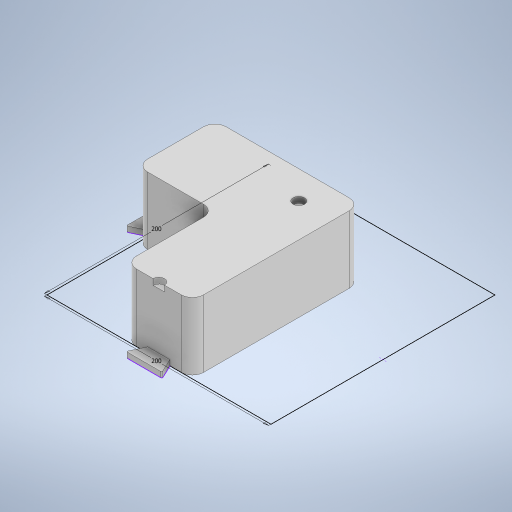
# Autodesk Inventor part: Area øv1
Saved by Autodesk Inventor 2024 (Build 280153000, 153)
## iProperties
Created: 2024-03-01
Part Number: Area øv1
Material: Generic
Document SubType Name: Modeling
Designer: laura
Density: 1 g/cm^3
Appearance: Default
Author: laura
Autodesk Inventor part; units mm, degrees
ref_plane "YZ Plane" through (0, 0, 0) normal (1, 0, 0) x (0, 1, 0)
ref_plane "XZ Plane" through (0, 0, 0) normal (0, 1, 0) x (-1, 0, 0)
ref_plane "XY Plane" through (0, 0, 0) normal (0, 0, 1) x (1, 0, 0)
sketch "Sketch1" plane through (0, 0, 0) normal (0, 1, 0) x (-1, 0, 0)
  line L0 (0, 0) -> (200, 0)
  line L1 (200, 0) -> (200, 200)
  line L2 (200, 200) -> (0, 200)
  line L3 (0, 200) -> (0, 0)
  line L4 (110, 199.8) -> (110, 213.2303) construction
  line L5 (100, 213.1946) -> (114.7696, 213.1946)
  arc A0 (115.4946, 212.0565) -> (114.7696, 213.1946) centre (114.7696, 212.3946) ccw
  line L6 (115.4946, 212.0565) -> (109.8726, 200)
  line L7 (109.8726, 200) -> (90.1274, 200)
  line L8 (90.1274, 200) -> (84.5054, 212.0565)
  arc A1 (85.2304, 213.1946) -> (84.5054, 212.0565) centre (85.2304, 212.3946) ccw
  line L9 (85.2304, 213.1946) -> (100, 213.1946)
  line L10 (200, 89.8726) -> (200, 110.1274)
  line L11 (200, 90.1274) -> (200, 109.8726)
  line L12 (200, 109.8726) -> (212.0565, 115.4946)
  arc A2 (213.1946, 114.7696) -> (212.0565, 115.4946) centre (212.3946, 114.7696) ccw
  line L13 (213.1946, 114.7696) -> (213.1946, 100)
  line L14 (199.8, 90) -> (213.2303, 90) construction
  line L15 (212.0565, 84.5054) -> (200, 90.1274)
  line L16 (213.1946, 100) -> (213.1946, 85.2304)
  arc A3 (212.0565, 84.5054) -> (213.1946, 85.2304) centre (212.3946, 85.2304) ccw
  point P0 (0, 100)
  point P1 (0, 100)
  point P2 (0, 100)
  point P3 (0, 100)
  point P4 (100, 200)
  point P5 (100, 200)
  point P6 (100, 200)
  point P7 (100, 200)
  point P8 (100, 200)
  point P9 (100, 200)
  point P10 (200, 100)
  point P11 (200, 100)
  point P12 (200, 100)
  point P13 (200, 100)
  point P14 (200, 100)
  point P15 (200, 100)
  point P16 (200, 100)
  point P17 (200, 100)
  point P18 (200, 100)
  point P19 (200, 100)
  dimension "d0" = 200
  dimension "d1" = 200
  constraints: 34 end point, 8 point on circle, 4 centre point, 4 midpoint, 2 parallel, 1 horizontal, 1 perpendicular
  measures "d0" distance of L2.end L1.end
  measures "d1" distance of L1.end L0.end
extrude "Extrusion1" add sketch "Sketch1" along normal blind 60 contours L3 L2 L1 L0
extrude "Extrusion3" add sketch "Sketch1" along normal blind 4.8 contours L8 A1 L9 L5 A0 L6 L2 | L1 L12 A2 L13 L16 A3 L15
sketch "Sketch2" plane through (0, 60, 0) normal (0, 1, 0) x (1, 0, 0)
  line L0 (0, 0) -> (-200, 0) projected
  circle A0 centre (-100, -75) radius 5.1
  circle A1 centre (-100, -200) radius 5.1
  dimension "d11" = 10.2
  dimension "d12" = 10.2
  constraints: 2 centre point
  measures "d11" diameter of A0
  measures "d12" diameter of A1
extrude "Extrusion4" cut sketch "Sketch2" against normal blind 5.2
sketch "Sketch3" plane through (0, 60, 0) normal (0, 1, 0) x (1, 0, 0)
  line L0 (0, -200) -> (0, 0) projected
  line L1 (-94.9, -200) -> (0, -200) projected
  line L2 (0, 0) -> (-70, 0)
  line L3 (-70, 0) -> (-70, -200)
  line L4 (-70, -200) -> (0, -200)
  line L5 (0, -200) -> (0, 0)
  line L6 (-200, 0) -> (-200, -200) projected
  line L7 (-200, 0) -> (0, 0)
  line L8 (0, 0) -> (0, -50)
  line L9 (0, -50) -> (-200, -50)
  line L10 (-200, -50) -> (-200, 0)
  line L11 (-200, -200) -> (-130, -200)
  line L12 (-130, -200) -> (-130, -120)
  line L13 (-130, -120) -> (-200, -120)
  line L14 (-200, -120) -> (-200, -200)
  point P0 (-70, -50)
  dimension "d17" = 70
  dimension "d18" = 50
  dimension "d19" = 70
  dimension "d20" = 80
  constraints: 24 end point, 6 parallel, 3 horizontal, 3 perpendicular, 2 point on line
  measures "d17" distance of L4.end L3.end
  measures "d18" distance of L7.end L8.end
  measures "d19" distance of L13.end L12.end
  measures "d20" distance of L12.end L11.end
extrude "Extrusion6" cut sketch "Sketch3" against normal blind 60
fillet "Fillet1" radius 10 6 edges at (-70, 30, 50) (-200, 30, 50) (-70, 30, 200) (-200, 30, 120) (-130, 30, 120) (-130, 30, 200)
body "Solid1"
